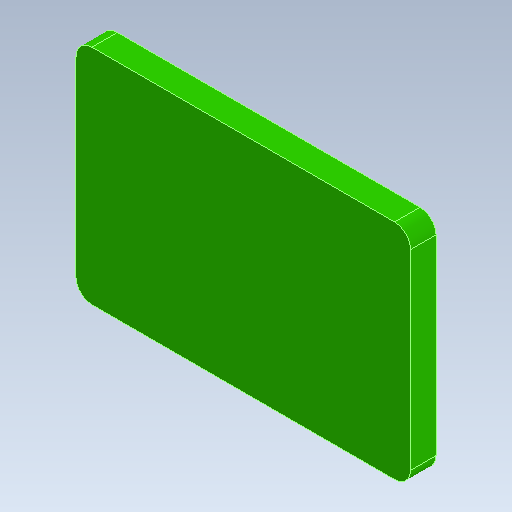
# Autodesk Inventor part: HDMI_ADAPTER_PCB
Saved by Autodesk Inventor 2021 (Build 250183000, 183)
## iProperties
Created: 2020-07-10
Part Number: HDMI_ADAPTER_PCB
Material: Generic
Document SubType Name: Modeling
Designer: lgnds
Density: 1 g/cm^3
Appearance: Default
Author: lgnds
Autodesk Inventor part; units mm, degrees
ref_plane "YZ Plane" through (0, 0, 0) normal (1, 0, 0) x (0, 1, 0)
ref_plane "XZ Plane" through (0, 0, 0) normal (0, 1, 0) x (-1, 0, 0)
ref_plane "XY Plane" through (0, 0, 0) normal (0, 0, 1) x (1, 0, 0)
sketch "Sketch1" plane through (0, 0, 0) normal (0, 0, 1) x (1, 0, 0)
  line L0 (-10.5, -7) -> (10.5, -7)
  line L1 (10.5, -7) -> (10.5, 7)
  line L2 (10.5, 7) -> (-10.5, 7)
  line L3 (-10.5, 7) -> (-10.5, -7)
  line L4 (-10.5, -7) -> (10.5, 7) construction
  line L5 (10.5, -7) -> (-10.5, 7) construction
  point P0 (0, 0)
  dimension "d0" = 21
  dimension "d1" = 14
  constraints: 12 end point, 2 midpoint, 2 parallel, 1 horizontal, 1 perpendicular
  measures "d0" distance of L1.end L2.end
  measures "d1" distance of L0.end L1.end
extrude "Extrusion1" add sketch "Sketch1" along normal blind 1.6
fillet "Fillet1" radius 1 4 edges at (10.5, 7, 0.8) (10.5, -7, 0.8) (-10.5, -7, 0.8) (-10.5, 7, 0.8)
sketch "HDMI_ADAPTER_PCB_OUTLINE" plane through (0, 0, 1.6) normal (0, 0, 1) x (1, 0, 0)
  line L0 (6.5, 2.68) -> (6.5, -0.32) projected
  line L1 (6.2, -0.32) -> (6.2, 2.68) projected
  line L2 (6.2, 2.68) -> (6.5, 2.68) projected
  line L3 (6.5, -0.32) -> (6.2, -0.32) projected
  line L4 (-6.5, -0.32) -> (-6.5, 2.68) projected
  line L5 (-6.2, 2.68) -> (-6.2, -0.32) projected
  line L6 (-6.5, 2.68) -> (-6.2, 2.68) projected
  line L7 (-6.2, -0.32) -> (-6.5, -0.32) projected
  circle A0 centre (-6.35, 1.18) radius 1.5
  circle A1 centre (6.35, 1.18) radius 1.5
  arc A2 (-9.5, 7) -> (-10.5, 6) centre (-9.5, 6) ccw projected
  line L8 (-10.5, 6) -> (-10.5, -6) projected
  arc A3 (-10.5, -6) -> (-9.5, -7) centre (-9.5, -6) ccw projected
  line L9 (-9.5, -7) -> (9.5, -7) projected
  arc A4 (9.5, -7) -> (10.5, -6) centre (9.5, -6) ccw projected
  line L10 (10.5, -6) -> (10.5, 6) projected
  arc A5 (10.5, 6) -> (9.5, 7) centre (9.5, 6) ccw projected
  line L11 (9.5, 7) -> (-9.5, 7) projected
  point P0 (0, 0)
  dimension "d5" = 0.3
  dimension "d6" = 0.15
  dimension "d7" = 0.15
  constraints: 4 tangent, 2 centre point
  measures "d5" distance between parallel lines of L5 L4
  measures "d6" distance from line of L4 A0.centre
  measures "d7" distance from line of L0 A1.centre
equation "\"d6\" = 0.5 * d5"
equation "\"d7\" = d6"
body "Solid1"
